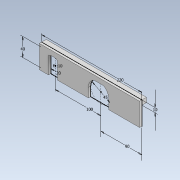
# Autodesk Inventor part: Gabel_Positionierung_Schablone
Saved by Autodesk Inventor 2022 (Build 260153000, 153)
## iProperties
Created: 2022-09-06
Part Number: Gabel_Positionierung_Schablone
Material: Generisch
Document SubType Name: Modeling
Designer: alexw
Density: 1 g/cm^3
Appearance: Vorgabe
Author: alexw
Autodesk Inventor part; units mm, degrees
ref_plane "YZ Plane" through (0, 0, 0) normal (1, 0, 0) x (0, 1, 0)
ref_plane "XZ Plane" through (0, 0, 0) normal (0, 1, 0) x (-1, 0, 0)
ref_plane "XY Plane" through (0, 0, 0) normal (0, 0, 1) x (1, 0, 0)
sketch "Skizze1" plane through (0, 0, 0) normal (0, 0, 1) x (1, 0, 0)
  line L0 (0, 0) -> (220, 0)
  line L1 (220, 0) -> (220, 50)
  line L2 (220, 50) -> (0, 50)
  line L3 (0, 50) -> (0, 0)
  line L4 (0, 50) -> (220, 50)
  line L5 (220, 50) -> (220, 40)
  line L6 (220, 40) -> (0, 40)
  line L7 (0, 40) -> (0, 50)
  line L8 (130, 0) -> (130, 40) construction
  line L9 (30, 0) -> (30, 40) construction
  circle A0 centre (130, 20) radius 22.5 construction
  circle A1 centre (30, 20) radius 20 construction
  line L10 (20, 0) -> (20, 37.3205)
  line L11 (40, 0) -> (40, 37.3205)
  arc A2 (40, 37.3205) -> (20, 37.3205) centre (30, 20) ccw
  arc A3 (20, 2.6795) -> (40, 2.6795) centre (30, 20) ccw construction
  line L12 (107.5, 20) -> (107.5, 0)
  line L13 (152.5, 20) -> (152.5, 0)
  arc A4 (119.6922, 40) -> (107.5, 20) centre (130, 20) ccw
  arc A5 (152.5, 20) -> (140.3078, 40) centre (130, 20) ccw
  point P0 (0, 40)
  dimension "d0" = 10
  dimension "d1" = 100
  dimension "d2" = 90
  dimension "d3" = 220
  dimension "d4" = 40
  dimension "d5" = 45
  dimension "d6" = 20
  dimension "d7" = 10
  constraints: 28 end point, 18 point on circle, 13 point on line, 6 centre point, 6 perpendicular, 5 parallel, 5 tangent, 2 concentric, 2 horizontal, 2 midpoint, 1 vertical
  measures "d0" distance between parallel lines of L2 L6
  measures "d1" distance between parallel lines of L8 L9
  measures "d2" distance between parallel lines of L1 L8
  measures "d3" distance between parallel lines of L1 L3
  measures "d4" distance between parallel lines of L0 L6
  measures "d5" diameter of A0
  measures "d6" distance between parallel lines of L11 L10
  measures "d7" distance between parallel lines of L11 L9
extrude "Extrusion1" add sketch "Skizze1" along normal blind 5 contours L3 L6 A2 L10 L0 | L3 L2 L1 L6 | L11 A2 L6 A4 L12 L0 | L13 A5 L6 L1 L0
extrude "Extrusion2" add sketch "Skizze1" against normal blind 10 contours L3 L2 L1 L6
equation "\"d7\" = 0.5 * d6"
